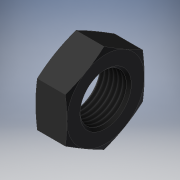
# Autodesk Inventor part: L073800800
Saved by Autodesk Inventor 2019 (Build 230136000, 136)
## iProperties
Created: 2023-02-15
Part Number: L073800800
Material: Generic
Catalog Web Link: www.cadenas.de
Description: SR Series Mounting Nut-Pneumatic Cylinder
Vendor: PARKERHANNIFIN
Document SubType Name: Modeling
Designer: psAdmin
Manufacturer: PARKERHANNIFIN
Mass: 3.16349 g
Surface Area: 18.3375 cm^2
Volume: 3.16349 cm^3
Density: 1 g/cm^3
Appearance: PSOLRGB-175-175-175
Category: PARTsolutions
Company: PARKERHANNIFIN
Title: L073800800
Author: Cadenas PARTsolutions
Comments: Pneumatic Cylinder
PSOL_IDENT_0: {$CADENAS_DATA/23d-libs/parkerpdn/actuators_cylinders/pneumatic_cylinders/accessories/sr_mounting_nu
PSOL_IDENT_1: t.prj},179 {VTYP=3D},{NB=L073800800},{LINA=L073800800},{NN=SR Series Mounting Nut},{DATE=26.07.2021
PSOL_IDENT_2: 05:25:38},{GEOMDATE=03.08.2017 08:20:29},{VERSION=},{LINEID=50},{WBVAR=MAT},{WBNUMERIC=}  {NB=L07380
PSOL_IDENT_3: 0800},{LINA=L073800800},{KT=DUMMY},{PN=L073800800},{PN1=L073800800},{PN2=L077170800},{BORE=3/4, 7/8,
PSOL_IDENT_4: 1-1/16},{MAT=},{MATVAL='' , 'Standard', 'S' , 'Stainless Steel'},{A=0.94},{B=0.38},{C=5/8-18},{THD=
PSOL_IDENT_5: 0.6250},{THDT=0.625}
NB: L073800800
NN: SR Series Mounting Nut
NT: Pneumatic Cylinder
NBSYN: $PN.
LINA: L073800800
CATALOG: Parker Pneumatic Division
PN: L073800800
BORE: 3/4, 7/8, 1-1/16
MAT: Standard
A: 0.94
B: 0.38
C: 5/8-18
SUPPLIER: PARKERHANNIFIN
ARTICLENO: L073800800
BOMINFO: L073800800
CREATOR: CADENAS GmbH
Autodesk Inventor part; units mm, degrees
sketch "Sketch_1" plane through (0, 0, 0) normal (0, 0, 1) x (1, 0, 0)
  line L0 (9.652, 0) -> (0, 0)
  line L1 (0, 0) -> (0, 11.938)
  line L2 (0, 11.938) -> (0.9596, 15.5194)
  line L3 (0.9596, 15.5194) -> (8.6924, 15.5194)
  line L4 (8.6924, 15.5194) -> (9.652, 11.938)
  line L5 (9.652, 11.938) -> (9.652, 0)
  line L6 (9.652, 0) -> (0, 0)
  constraints: 14 end point
revolve "Revolution1" add sketch "Sketch_1" angle 360 about axis through (9.652, 0, 0) along (1, 0, 0)
sketch "Sketch_2" plane through (0, 0, 0) normal (1, 0, 0) x (0, 1, 0)
  line L0 (-23.876, 23.876) -> (-23.876, -23.876)
  line L1 (-23.876, -23.876) -> (23.876, -23.876)
  line L2 (23.876, -23.876) -> (23.876, 23.876)
  line L3 (23.876, 23.876) -> (-23.876, 23.876)
  line L4 (-6.8924, 11.938) -> (-13.7848, 0)
  line L5 (-13.7848, 0) -> (-6.8924, -11.938)
  line L6 (-6.8924, -11.938) -> (6.8924, -11.938)
  line L7 (6.8924, -11.938) -> (13.7848, 0)
  line L8 (13.7848, 0) -> (6.8924, 11.938)
  line L9 (6.8924, 11.938) -> (-6.8924, 11.938)
  constraints: 20 end point
extrude "Extrusion1" cut sketch "Sketch_2" along normal blind 9.652
sketch "Sketch_3" plane through (0, 0, 0) normal (0, 0, 1) x (1, 0, 0)
  line L0 (9.652, 0) -> (0, 0)
  line L1 (0, 0) -> (0, 7.9375)
  line L2 (0, 7.9375) -> (0.7633, 7.1742)
  line L3 (0.7633, 7.1742) -> (8.8887, 7.1742)
  line L4 (8.8887, 7.1742) -> (9.652, 7.9375)
  line L5 (9.652, 7.9375) -> (9.652, 0)
  line L6 (9.652, 0) -> (0, 0)
  constraints: 14 end point
revolve "Revolution2" cut sketch "Sketch_3" angle 360 about axis through (9.652, 0, 0) along (1, 0, 0)
thread "Thread1" size "5/8-18 UNF" class "2B" standard "ANSI Unified Screw Threads" full length
ref_plane "c_XY" through (9.652, 0, 0) normal (1, 0, 0) x (0, 0, -1)
ref_plane "c_YZ" through (9.652, 0, 0) normal (0, 0, -1) x (0, 1, 0)
ref_plane "c_ZX" through (9.652, 0, 0) normal (0, 1, 0) x (1, 0, 0)
ref_plane "kb_XY" through (4.826, -11.938, 0) normal (0, 0, 1) x (1, 0, 0)
ref_plane "kb_YZ" through (4.826, -11.938, 0) normal (1, 0, 0) x (0, 1, 0)
ref_plane "kb_ZX" through (4.826, -11.938, 0) normal (0, 1, 0) x (0, 0, 1)
ref_plane "nut_XY" through (0, 0, 0) normal (1, 0, 0) x (0, 0, -1)
ref_plane "nut_YZ" through (0, 0, 0) normal (0, 0, -1) x (0, 1, 0)
ref_plane "nut_ZX" through (0, 0, 0) normal (0, 1, 0) x (1, 0, 0)
body "Solid1"
